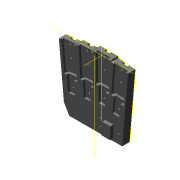
# Autodesk Inventor part: empty
Saved by Autodesk Inventor 2014 (Build 180170000, 170)
## iProperties
Created: 2015-04-13
Part Number: empty
Material: Generic
Document SubType Name: Modeling
Designer: Martin
Density: 1 g/cm^3
Appearance: Default
Author: Martin
Autodesk Inventor part; units mm, degrees
sketch "block_finger_attachment" plane through (0, 0, 0) normal (0, 0, 1) x (1, 0, 0)
  circle A0 centre (0, 0) radius 1.75
  circle A1 centre (0, -15) radius 1.75
  circle A2 centre (0, -46.8) radius 1.75
  line L0 (-8.5, -52.8) -> (8.5, -52.8)
  line L1 (8.5, -52.8) -> (8.5, 2.75)
  line L2 (8.5, 2.75) -> (-8.5, 2.75)
  line L3 (-8.5, 2.75) -> (-8.5, -52.8)
  line L4 (-8.5, -52.8) -> (8.5, 2.75) construction
  line L5 (8.5, -52.8) -> (-8.5, 2.75) construction
  line L6 (0, 2.75) -> (0, -52.8) construction
  line L7 (-8.5, -34.3) -> (8.5, -34.3)
  line L8 (-8.5, -31.5) -> (8.5, -31.5)
  line L9 (-4, -34.3) -> (-4, -52.8)
  line L10 (4, -34.3) -> (4, -52.8)
  line L11 (-8.5, -36.8) -> (8.5, -36.8) construction
  point P0 (0, -23.8707)
  point P1 (0, -25.025)
  dimension "d24" = 3.5
  dimension "d26" = 31.8
  dimension "d28" = 6
  dimension "d30" = 17
  dimension "d49" = 2.8
  dimension "d50" = 18.5
  dimension "d68" = 8
  dimension "d69" = 2.75
  dimension "d70" = 15
  dimension "d87" = 16
  measures "d24" diameter of A0
  measures "d26" distance of A2.centre A1.centre
  measures "d28" distance from line of L0 A2.centre
  measures "d30" distance of L0.start L0.end
  measures "d49" distance between parallel lines of L7 L8
  measures "d50" distance between parallel lines of L0 L7
  measures "d68" distance between parallel lines of L10 L9
  measures "d69" distance from line of L2 A0.centre
  measures "d70" distance of A0.centre A1.centre
  measures "d87" distance between parallel lines of L11 L0
sketch "block_finger_cutway" plane through (0, 0, 0) normal (0, 0, 1) x (1, 0, 0)
  circle A0 centre (0, 0) radius 1.75 construction
  circle A1 centre (0, -15) radius 1.75 construction
  circle A2 centre (0, -46.8) radius 1.75 construction
  line L0 (-8.5, -52.8) -> (8.5, -52.8) construction
  line L1 (8.5, -52.8) -> (8.5, 2.75) construction
  line L2 (8.5, 2.75) -> (-8.5, 2.75) construction
  line L3 (-8.5, 2.75) -> (-8.5, -52.8) construction
  line L4 (-8.5, -52.8) -> (8.5, 2.75) construction
  line L5 (8.5, -52.8) -> (-8.5, 2.75) construction
  line L6 (0, 2.75) -> (0, -52.8) construction
  line L7 (-8.5, -34.3) -> (8.5, -34.3) construction
  line L8 (-8.5, -31.5) -> (8.5, -31.5) construction
  line L9 (-4.5, -34.3) -> (-4.5, -52.8)
  line L10 (4.5, -34.3) -> (4.5, -52.8)
  line L11 (-8.5, -36.8) -> (8.5, -36.8) construction
  line L12 (-4.5, -52.8) -> (4.5, -52.8)
  line L13 (-4.5, -34.3) -> (-8, -34.3)
  line L14 (-8, -34.3) -> (-8, 2.75)
  line L15 (-8, 2.75) -> (8, 2.75)
  line L16 (8, 2.75) -> (8, -34.3)
  line L17 (4.5, -34.3) -> (8, -34.3)
  line L18 (4.5, -37.3) -> (8.5, -37.3)
  line L19 (8.5, -37.3) -> (8.5, -25.8)
  line L20 (8.5, -25.8) -> (8, -25.8)
  line L21 (-4.5, -52.8) -> (4.5, -52.8)
  line L22 (4.5, -52.8) -> (4.5, -53.8)
  line L23 (4.5, -53.8) -> (-4.5, -53.8)
  line L24 (-4.5, -53.8) -> (-4.5, -52.8)
  point P0 (0, -23.8707)
  point P1 (0, -25.025)
  dimension "d109" = 3.5
  dimension "d110" = 31.8
  dimension "d111" = 6
  dimension "d112" = 17
  dimension "d113" = 2.8
  dimension "d114" = 18.5
  dimension "d115" = 9
  dimension "d116" = 2.75
  dimension "d117" = 15
  dimension "d118" = 16
  dimension "d119" = 0.5
  dimension "d122" = 11.5
  dimension "d123" = 3
  dimension "d124" = 0.5
  dimension "d136" = 1
  measures "d109" diameter of A0
  measures "d110" distance of A2.centre A1.centre
  measures "d111" distance from line of L0 A2.centre
  measures "d112" distance of L0.start L0.end
  measures "d113" distance between parallel lines of L7 L8
  measures "d114" distance between parallel lines of L0 L7
  measures "d115" distance between parallel lines of L10 L9
  measures "d116" distance from line of L2 A0.centre
  measures "d117" distance of A0.centre A1.centre
  measures "d118" distance between parallel lines of L11 L0
  measures "d119" distance between parallel lines of L3 L14
  measures "d122" distance of L18.end L19.end
  measures "d123" distance between parallel lines of L7 L18
  measures "d124" distance between parallel lines of L16 L19
  measures "d136" distance between parallel lines of L0 L23
sketch "sk_main" plane through (0, 0, 0) normal (0, 1, 0) x (-1, 0, 0)
  line L0 (74.2951, 0) -> (-52.28, 0) projected
  line L1 (0, -108) -> (0, 18) projected
  line L2 (0, -3) -> (-23.2397, -3) construction
  line L3 (-8.5, -55.55) -> (-10.1097, -55.55) construction
  line L4 (0, -4) -> (22.6679, -4) construction
  line L5 (8.5, -55.55) -> (10.9991, -55.55) construction
  line L6 (0, -8) -> (45.2636, -8) construction
  line L7 (27.7608, -59.9653) -> (31.7206, -59.9653) construction
  line L8 (36.8027, -7.1853) -> (33.9128, -6.907)
  line L9 (33.9128, -6.907) -> (34.0419, -4.7972)
  line L10 (14.1837, -3.4811) -> (11.345, -3.293)
  line L11 (11.345, -3.293) -> (11.345, 0)
  line L12 (-14.772, -2.2592) -> (-11.642, -1.9853)
  line L13 (-11.642, -1.9853) -> (-11.642, 0)
  line L14 (56.2129, -9.0543) -> (49.5831, -77.9074)
  line L15 (42.6015, -90) -> (-26.6702, -90)
  line L16 (-26.6702, -90) -> (-34.1978, -3.9587)
  line L17 (-34.1978, -3.9587) -> (-31.7073, -3.7408)
  line L18 (49.5831, -77.9074) -> (42.6015, -90)
  line L19 (-8.5, 0) -> (-11.642, 0)
  line L20 (11.345, 0) -> (8.5, 0)
  line L21 (31.152, -4.5189) -> (34.0419, -4.7972)
  line L22 (53.7244, -8.8147) -> (56.2129, -9.0543)
  line L23 (33.9128, -6.907) -> (56.2129, -9.0543)
  line L24 (34.0419, -4.7972) -> (11.345, -3.293)
  line L25 (11.345, 0) -> (-11.642, 0)
  line L26 (-11.642, -1.9853) -> (-34.1978, -3.9587)
  circle A0 centre (-23, -5.7395) radius 1.75
  circle A1 centre (-21.6927, -20.6825) radius 1.75
  circle A2 centre (-18.9211, -52.3614) radius 1.75
  line L27 (-26.8658, -59.0794) -> (-9.9305, -57.5978)
  line L28 (-9.9305, -57.5978) -> (-14.772, -2.2592)
  line L29 (-14.772, -2.2592) -> (-31.7073, -3.7408)
  line L30 (-31.7073, -3.7408) -> (-26.8658, -59.0794)
  line L31 (-26.8658, -59.0794) -> (-14.772, -2.2592) construction
  line L32 (-9.9305, -57.5978) -> (-31.7073, -3.7408) construction
  line L33 (-23.2397, -3) -> (-18.3982, -58.3386) construction
  line L34 (-28.4782, -40.6498) -> (-11.5429, -39.1682)
  line L35 (-28.7222, -37.8605) -> (-11.7869, -36.3788)
  line L36 (-23.9953, -40.2576) -> (-22.383, -58.6872)
  line L37 (-16.0258, -39.5604) -> (-14.4134, -57.99)
  line L38 (-28.2603, -43.1403) -> (-11.325, -41.6587) construction
  circle A3 centre (0, -2.75) radius 1.75
  circle A4 centre (0, -17.75) radius 1.75
  circle A5 centre (0, -49.55) radius 1.75
  line L39 (-8.5, -55.55) -> (8.5, -55.55)
  line L40 (8.5, -55.55) -> (8.5, 0)
  line L41 (8.5, 0) -> (-8.5, 0)
  line L42 (-8.5, 0) -> (-8.5, -55.55)
  line L43 (-8.5, -55.55) -> (8.5, 0) construction
  line L44 (8.5, -55.55) -> (-8.5, 0) construction
  line L45 (0, 0) -> (0, -55.55) construction
  line L46 (-8.5, -37.05) -> (8.5, -37.05)
  line L47 (-8.5, -34.25) -> (8.5, -34.25)
  line L48 (-4, -37.05) -> (-4, -55.55)
  line L49 (4, -37.05) -> (4, -55.55)
  line L50 (-8.5, -39.55) -> (8.5, -39.55) construction
  circle A6 centre (22.5, -6.7449) radius 1.75
  circle A7 centre (21.5843, -21.7169) radius 1.75
  circle A8 centre (19.6429, -53.4576) radius 1.75
  line L51 (10.7925, -58.9275) -> (27.7608, -59.9653)
  line L52 (27.7608, -59.9653) -> (31.152, -4.5189)
  line L53 (31.152, -4.5189) -> (14.1837, -3.4811)
  line L54 (14.1837, -3.4811) -> (10.7925, -58.9275)
  line L55 (10.7925, -58.9275) -> (31.152, -4.5189) construction
  line L56 (27.7608, -59.9653) -> (14.1837, -3.4811) construction
  line L57 (22.6679, -4) -> (19.2766, -59.4464) construction
  line L58 (11.9219, -40.462) -> (28.8902, -41.4998)
  line L59 (12.0928, -37.6672) -> (29.0611, -38.705)
  line L60 (16.4135, -40.7367) -> (15.2841, -59.2022)
  line L61 (24.3986, -41.2251) -> (23.2692, -59.6906)
  line L62 (11.7693, -42.9573) -> (28.7376, -43.9951) construction
  circle A9 centre (45, -10.7373) radius 1.75
  circle A10 centre (43.5623, -25.6683) radius 1.75
  circle A11 centre (40.5144, -57.3219) radius 1.75
  line L63 (31.4785, -62.4796) -> (48.4002, -64.1089)
  line L64 (48.4002, -64.1089) -> (53.7244, -8.8147)
  line L65 (53.7244, -8.8147) -> (36.8027, -7.1853)
  line L66 (36.8027, -7.1853) -> (31.4785, -62.4796)
  line L67 (31.4785, -62.4796) -> (53.7244, -8.8147) construction
  line L68 (48.4002, -64.1089) -> (36.8027, -7.1853) construction
  line L69 (45.2636, -8) -> (39.9393, -63.2943) construction
  line L70 (33.2516, -44.0647) -> (50.1734, -45.6941)
  line L71 (33.52, -41.2776) -> (50.4417, -42.907)
  line L72 (37.7309, -44.496) -> (35.9578, -62.9109)
  line L73 (45.6941, -45.2628) -> (43.9209, -63.6776)
  line L74 (33.012, -46.5532) -> (49.9337, -48.1826) construction
  point P0 (0, 0)
  dimension "d32" = 23
  dimension "d37" = 22.5
  dimension "d41" = 22.5
  dimension "d31" = 5
  dimension "d33" = 3
  dimension "d34" = 1.6097
  dimension "d35" = 3.5
  dimension "d36" = 4
  dimension "d38" = 2.4991
  dimension "d39" = 5.5
  dimension "d40" = 8
  dimension "d42" = 3.9598
  dimension "d43" = 2.5
  dimension "d44" = 2.5
  dimension "d45" = 90
  constraints: 50 end point, 6 collinear, 6 parallel, 5 point on line, 4 perpendicular, 3 equal length, 1 vertical, 25 other
  measures "d33" distance between parallel lines of L0 L2
  measures "d34" distance of L3.start L3.end
  measures "d36" distance between parallel lines of L0 L4
  measures "d38" distance of L5.start L5.end
  measures "d40" distance between parallel lines of L0 L6
  measures "d42" distance of L7.start L7.end
  measures "d45" distance between parallel lines of L0 L15
extrude "ext_main" add sketch "sk_main" along normal blind 10 contours L11 L10 L54 L51 L52 L24 L9 L8 L66 L63 L64 L22 L14 L18 L15 L1 L39 L40 L0 | L40 L47 L1 A4 A3 L0 | L1 A3 A4 L47 L42 L0 | L40 L46 L1 L47 | L24 L52 L59 L54 | L42 L39 L1 L15 L16 L17 L30 L27 L28 L12 L13 L0 | L40 L39 L49 L46 | L1 L46 L42 L47 | L59 L52 L58 L54 | L49 L39 L1 A5 L46 | L1 A5 L39 L48 L46 | L58 L60 L51 L54 | L46 L48 L39 L42 | L52 L51 L61 L58 | L58 L61 L51 L60 | L28 L35 L30 L26 | L23 L64 L71 L66 | L28 L34 L30 L35 | L71 L64 L70 L66 | L28 L27 L37 L34 | L70 L72 L63 L66 | L34 L36 L27 L30 | L37 L27 L36 L34 | L64 L63 L73 L70 | L70 L73 L63 L72
ref_plane "plane_gear_4" through (-33.52, 0, -41.2776) normal (0.0958458, 0, -0.9953962) x (0, 1, 0)
ref_plane "plane_gear_3" through (-12.0928, 0, -37.6672) normal (0.0610485, 0, -0.9981348) x (0, 1, 0)
ref_plane "plane_gear_2" through (8.5, 0, -34.25) normal (0, 0, -1) x (-1, 0, 0)
ref_plane "plane_gear_1" through (28.7222, 0, -37.8605) normal (-0.0871557, 0, -0.9961947) x (0, -1, 0)
sketch "sk_cutways" plane through (0, 0, 0) normal (0, -1, 0) x (1, 0, 0)
  line L0 (0, -108) -> (0, 18) projected
  circle A0 centre (-45, -10.7373) radius 1.75 projected
  circle A1 centre (-43.5623, -25.6683) radius 1.75 projected
  circle A2 centre (-22.5, -6.7449) radius 1.75 projected
  circle A3 centre (-21.5843, -21.7169) radius 1.75 projected
  circle A4 centre (0, -17.75) radius 1.75 projected
  circle A5 centre (0, -2.75) radius 1.75 projected
  circle A6 centre (23, -5.7395) radius 1.75 projected
  circle A7 centre (21.6927, -20.6825) radius 1.75 projected
  circle A8 centre (-45, -10.7373) radius 1.75 construction
  circle A9 centre (-43.5623, -25.6683) radius 1.75 construction
  circle A10 centre (-40.5144, -57.3219) radius 1.75 construction
  line L1 (-48.4002, -64.1089) -> (-31.4785, -62.4796) construction
  line L2 (-31.4785, -62.4796) -> (-36.8027, -7.1853) construction
  line L3 (-36.8027, -7.1853) -> (-53.7244, -8.8147) construction
  line L4 (-53.7244, -8.8147) -> (-48.4002, -64.1089) construction
  line L5 (-48.4002, -64.1089) -> (-36.8027, -7.1853) construction
  line L6 (-31.4785, -62.4796) -> (-53.7244, -8.8147) construction
  line L7 (-45.2636, -8) -> (-39.9393, -63.2943) construction
  line L8 (-50.1734, -45.6941) -> (-33.2516, -44.0647) construction
  line L9 (-50.4417, -42.907) -> (-33.52, -41.2776) construction
  line L10 (-46.1918, -45.3107) -> (-44.4186, -63.7256)
  line L11 (-37.2332, -44.4481) -> (-35.4601, -62.863)
  line L12 (-49.9337, -48.1826) -> (-33.012, -46.5532) construction
  line L13 (-44.4186, -63.7256) -> (-35.4601, -62.863)
  line L14 (-46.1918, -45.3107) -> (-49.6757, -45.6462)
  line L15 (-49.6757, -45.6462) -> (-53.2267, -8.7668)
  line L16 (-53.2267, -8.7668) -> (-37.3004, -7.2332)
  line L17 (-37.3004, -7.2332) -> (-33.7493, -44.1127)
  line L18 (-37.2332, -44.4481) -> (-33.7493, -44.1127)
  line L19 (-36.9457, -47.4343) -> (-32.9641, -47.0509)
  line L20 (-32.9641, -47.0509) -> (-34.0663, -35.6039)
  line L21 (-34.0663, -35.6039) -> (-34.564, -35.6518)
  line L22 (-44.4186, -63.7256) -> (-35.4601, -62.863)
  line L23 (-35.4601, -62.863) -> (-35.3642, -63.8583)
  line L24 (-35.3642, -63.8583) -> (-44.3228, -64.721)
  line L25 (-44.3228, -64.721) -> (-44.4186, -63.7256)
  circle A11 centre (-22.5, -6.7449) radius 1.75 construction
  circle A12 centre (-21.5843, -21.7169) radius 1.75 construction
  circle A13 centre (-19.6429, -53.4576) radius 1.75 construction
  line L26 (-27.7608, -59.9653) -> (-10.7925, -58.9275) construction
  line L27 (-10.7925, -58.9275) -> (-14.1837, -3.4811) construction
  line L28 (-14.1837, -3.4811) -> (-31.152, -4.5189) construction
  line L29 (-31.152, -4.5189) -> (-27.7608, -59.9653) construction
  line L30 (-27.7608, -59.9653) -> (-14.1837, -3.4811) construction
  line L31 (-10.7925, -58.9275) -> (-31.152, -4.5189) construction
  line L32 (-22.6679, -4) -> (-19.2766, -59.4464) construction
  line L33 (-28.8902, -41.4998) -> (-11.9219, -40.462) construction
  line L34 (-29.0611, -38.705) -> (-12.0928, -37.6672) construction
  line L35 (-24.8976, -41.2556) -> (-23.7682, -59.7211)
  line L36 (-15.9144, -40.7062) -> (-14.785, -59.1717)
  line L37 (-28.7376, -43.9951) -> (-11.7693, -42.9573) construction
  line L38 (-23.7682, -59.7211) -> (-14.785, -59.1717)
  line L39 (-24.8976, -41.2556) -> (-28.3911, -41.4693)
  line L40 (-28.3911, -41.4693) -> (-30.653, -4.4884)
  line L41 (-30.653, -4.4884) -> (-14.6828, -3.5116)
  line L42 (-14.6828, -3.5116) -> (-12.421, -40.4925)
  line L43 (-15.9144, -40.7062) -> (-12.421, -40.4925)
  line L44 (-15.7313, -43.7006) -> (-11.7387, -43.4564)
  line L45 (-11.7387, -43.4564) -> (-12.4408, -31.9778)
  line L46 (-12.4408, -31.9778) -> (-12.9399, -32.0084)
  line L47 (-23.7682, -59.7211) -> (-14.785, -59.1717)
  line L48 (-14.785, -59.1717) -> (-14.724, -60.1698)
  line L49 (-14.724, -60.1698) -> (-23.7072, -60.7192)
  line L50 (-23.7072, -60.7192) -> (-23.7682, -59.7211)
  circle A14 centre (0, -2.75) radius 1.75 construction
  circle A15 centre (0, -17.75) radius 1.75 construction
  circle A16 centre (0, -49.55) radius 1.75 construction
  line L51 (-8.5, -55.55) -> (8.5, -55.55) construction
  line L52 (8.5, -55.55) -> (8.5, 0) construction
  line L53 (8.5, 0) -> (-8.5, 0) construction
  line L54 (-8.5, 0) -> (-8.5, -55.55) construction
  line L55 (-8.5, -55.55) -> (8.5, 0) construction
  line L56 (8.5, -55.55) -> (-8.5, 0) construction
  line L57 (0, 0) -> (0, -55.55) construction
  line L58 (-8.5, -37.05) -> (8.5, -37.05) construction
  line L59 (-8.5, -34.25) -> (8.5, -34.25) construction
  line L60 (-4.5, -37.05) -> (-4.5, -55.55)
  line L61 (4.5, -37.05) -> (4.5, -55.55)
  line L62 (-8.5, -39.55) -> (8.5, -39.55) construction
  line L63 (-4.5, -55.55) -> (4.5, -55.55)
  line L64 (-4.5, -37.05) -> (-8, -37.05)
  line L65 (-8, -37.05) -> (-8, 0)
  line L66 (-8, 0) -> (8, 0)
  line L67 (8, 0) -> (8, -37.05)
  line L68 (4.5, -37.05) -> (8, -37.05)
  line L69 (4.5, -40.05) -> (8.5, -40.05)
  line L70 (8.5, -40.05) -> (8.5, -28.55)
  line L71 (8.5, -28.55) -> (8, -28.55)
  line L72 (-4.5, -55.55) -> (4.5, -55.55)
  line L73 (4.5, -55.55) -> (4.5, -56.55)
  line L74 (4.5, -56.55) -> (-4.5, -56.55)
  line L75 (-4.5, -56.55) -> (-4.5, -55.55)
  circle A17 centre (23, -5.7395) radius 1.75 construction
  circle A18 centre (21.6927, -20.6825) radius 1.75 construction
  circle A19 centre (18.9211, -52.3614) radius 1.75 construction
  line L76 (9.9305, -57.5978) -> (26.8658, -59.0794) construction
  line L77 (26.8658, -59.0794) -> (31.7073, -3.7408) construction
  line L78 (31.7073, -3.7408) -> (14.772, -2.2592) construction
  line L79 (14.772, -2.2592) -> (9.9305, -57.5978) construction
  line L80 (9.9305, -57.5978) -> (31.7073, -3.7408) construction
  line L81 (26.8658, -59.0794) -> (14.772, -2.2592) construction
  line L82 (23.2397, -3) -> (18.3982, -58.3386) construction
  line L83 (11.5429, -39.1682) -> (28.4782, -40.6498) construction
  line L84 (11.7869, -36.3788) -> (28.7222, -37.8605) construction
  line L85 (15.5277, -39.5168) -> (13.9153, -57.9464)
  line L86 (24.4934, -40.3012) -> (22.8811, -58.7308)
  line L87 (11.325, -41.6587) -> (28.2603, -43.1403) construction
  line L88 (13.9153, -57.9464) -> (22.8811, -58.7308)
  line L89 (15.5277, -39.5168) -> (12.041, -39.2118)
  line L90 (12.041, -39.2118) -> (15.2701, -2.3028)
  line L91 (15.2701, -2.3028) -> (31.2092, -3.6972)
  line L92 (31.2092, -3.6972) -> (27.9801, -40.6063)
  line L93 (24.4934, -40.3012) -> (27.9801, -40.6063)
  line L94 (24.232, -43.2898) -> (28.2167, -43.6384)
  line L95 (28.2167, -43.6384) -> (29.219, -32.1822)
  line L96 (29.219, -32.1822) -> (28.7209, -32.1386)
  line L97 (13.9153, -57.9464) -> (22.8811, -58.7308)
  line L98 (22.8811, -58.7308) -> (22.7939, -59.727)
  line L99 (22.7939, -59.727) -> (13.8281, -58.9426)
  line L100 (13.8281, -58.9426) -> (13.9153, -57.9464)
  constraints: 9 other
extrude "ext_cut_linactcutways" cut sketch "sk_cutways" against normal blind 3 contours L74 L75 L63 L0 | L0 L63 L73 L74 | L63 L60 L64 L65 L66 L0 A5 A4 | L0 A4 A5 L66 L67 L68 L61 L63 | L61 L68 L67 L71 L70 L69 | L14 L15 L16 L17 L18 L11 L13 L10 | L13 L23 L24 L25 | L11 L18 L17 L21 L20 L19 | L39 L40 L41 L42 L43 L36 L38 L35 | L38 L48 L49 L50 | L36 L43 L42 L46 L45 L44 | L89 L90 L91 L92 L93 L86 L88 L85 | L88 L98 L99 L100 | L86 L93 L92 L96 L95 L94
chamfer "chamfer_linact_side" distance 1 angle 45 4 edges at (-33.5152, 0, -41.3274) (-12.0898, 0, -37.7171) (8.5, 0, -34.3) (28.7179, 0, -37.9103)
sketch "Sketch5" plane through (-33.52, 0, -41.2776) normal (0.0958458, 0, -0.9953962) x (0, 1, 0)
  line L0 (0, 0) -> (0, -17) projected
  line L1 (0, 0) -> (0, -17)
  line L2 (0, -17) -> (3, -17)
  line L3 (3, -17) -> (3, 0)
  line L4 (3, 0) -> (0, 0)
  arc A0 (3, -17) -> (3, 0) centre (-0.0208, -8.5) ccw
  line L5 (3, -8.5) -> (9, -8.5) construction
  point P0 (0, 37.322)
  dimension "d134" = 6
  dimension "d135" = 3
  constraints: 10 end point, 3 equal length, 3 point on circle, 1 centre point, 1 midpoint, 1 perpendicular
  measures "d134" distance of L5.start L5.end
  measures "d135" distance of L3.end L0.start
extrude "ext_cut_gear_4" cut sketch "Sketch5" along normal up to surface (2.8 mm away)
sketch "Sketch6" plane through (-12.0928, 0, -37.6672) normal (0.0610485, 0, -0.9981348) x (0, 1, 0)
  line L0 (0, 0) -> (0, -17) projected
  line L1 (0, -17) -> (0, 0)
  line L2 (0, 0) -> (3, 0)
  line L3 (3, 0) -> (3, -17)
  line L4 (3, -17) -> (0, -17)
  arc A0 (3, -17) -> (3, 0) centre (-0.0208, -8.5) ccw
  line L5 (3, -8.5) -> (9, -8.5)
  point P0 (0, 14.3698)
  dimension "d132" = 6
  dimension "d133" = 3
  constraints: 10 end point, 3 parallel, 3 point on circle, 1 centre point, 1 collinear, 1 midpoint, 1 perpendicular
  measures "d132" distance of L5.start L5.end
  measures "d133" distance of L0.start L2.end
extrude "ext_cut_gear_3" cut sketch "Sketch6" along normal up to surface (2.8 mm away)
sketch "Sketch7" plane through (8.5, 0, -34.25) normal (0, 0, -1) x (-1, 0, 0)
  line L0 (0, 0) -> (17, 0) projected
  line L1 (0, 0) -> (17, 0)
  line L2 (17, 0) -> (17, 3)
  line L3 (17, 3) -> (0, 3)
  line L4 (0, 3) -> (0, 0)
  arc A0 (17, 3) -> (0, 3) centre (8.5, -0.0208) ccw
  line L5 (8.5, 9) -> (8.5, 3) construction
  point P0 (8.5, 0)
  dimension "d130" = 6
  dimension "d131" = 3
  constraints: 10 end point, 3 equal length, 3 point on circle, 1 centre point, 1 midpoint, 1 perpendicular
  measures "d130" distance of L5.start L5.end
  measures "d131" distance of L0.end L2.end
extrude "ext_cut_gear_2" cut sketch "Sketch7" along normal up to surface (2.8 mm away)
sketch "Sketch8" plane through (28.7222, 0, -37.8605) normal (-0.0871557, 0, -0.9961947) x (0, -1, 0)
  line L0 (0, 0) -> (0, 17) projected
  line L1 (0, 17) -> (0, 0)
  line L2 (0, 0) -> (-3, 0)
  line L3 (-3, 0) -> (-3, 17)
  line L4 (-3, 17) -> (0, 17)
  arc A0 (-3, 17) -> (-3, 0) centre (0.0208, 8.5) ccw
  line L5 (-9, 8.5) -> (-3, 8.5) construction
  point P0 (0, 31.9127)
  dimension "d128" = 3
  dimension "d129" = 6
  constraints: 10 end point, 3 equal length, 3 point on circle, 1 centre point, 1 midpoint, 1 perpendicular
  measures "d128" distance of L3.end L0.end
  measures "d129" distance of L5.start L5.end
extrude "ext_cut_gear_1" cut sketch "Sketch8" along normal up to surface (2.8 mm away)
sketch "sk_thumb_axis" plane through (0, 0, 0) normal (0, 0, 1) x (1, 0, 0)
  line L0 (-2, 0) -> (12, 0) projected
  line L1 (0, -24) -> (0, 4) projected
  point P0 (0, 0)
  point P1 (10, -20)
  dimension "d66" = 20
  dimension "d67" = 10
  measures "d66" distance from line of L0 point (10, -20)
  measures "d67" distance from line of L1 point (10, -20)
ref_plane "plane_thumblinact" through (-9, 0, 0) normal (1, 0, 0) x (0, 1, 0)
sketch "Sketch9" plane through (0, 10, 0) normal (0, 1, 0) x (1, 0, 0)
  circle A0 centre (-40.5144, 57.3219) radius 1.75 projected
  circle A1 centre (-43.5623, 25.6683) radius 1.75 projected
  circle A2 centre (-45, 10.7373) radius 1.75 projected
  circle A3 centre (0, 49.55) radius 1.75 projected
  circle A4 centre (0, 17.75) radius 1.75 projected
  circle A5 centre (0, 2.75) radius 1.75 projected
  circle A6 centre (18.9211, 52.3614) radius 1.75 projected
  circle A7 centre (21.6927, 20.6825) radius 1.75 projected
  circle A8 centre (23, 5.7395) radius 1.75 projected
  circle A9 centre (-19.6429, 53.4576) radius 1.75 projected
  circle A10 centre (-21.5843, 21.7169) radius 1.75 projected
  circle A11 centre (-22.5, 6.7449) radius 1.75 projected
  line L0 (11.642, 1.9853) -> (34.1978, 3.9587) projected
  line L1 (-56.2129, 9.0543) -> (-33.9128, 6.907) projected
  line L2 (-34.0419, 4.7972) -> (-11.345, 3.293) projected
  line L3 (-11.345, 0) -> (11.642, 0) projected
  circle A12 centre (-40.5144, 57.3219) radius 3.25
  circle A13 centre (-19.6429, 53.4576) radius 3.25
  circle A14 centre (0, 49.55) radius 3.25
  circle A15 centre (18.9211, 52.3614) radius 3.25
  circle A16 centre (21.6927, 20.6825) radius 3.25
  circle A17 centre (23, 5.7395) radius 3.25
  circle A18 centre (0, 17.75) radius 3.25
  circle A19 centre (-21.5843, 21.7169) radius 3.25
  circle A20 centre (-22.5, 6.7449) radius 3.25
  circle A21 centre (0, 2.75) radius 3.25
  circle A22 centre (-43.5623, 25.6683) radius 3.25
  circle A23 centre (-45, 10.7373) radius 3.25
  line L4 (-48.4986, 8.3115) -> (-48.235, 11.0488)
  line L5 (-42.0285, 7.6885) -> (-41.765, 10.4258)
  line L6 (-25.9219, 4.259) -> (-25.7429, 6.9598)
  line L7 (-19.4361, 3.8292) -> (-19.2571, 6.53)
  line L8 (-3.25, 0) -> (-3.25, 2.75)
  line L9 (3.25, 0) -> (3.25, 2.75)
  line L10 (20.002, 2.7167) -> (19.7624, 5.4563)
  line L11 (26.4773, 3.2833) -> (26.2376, 6.0228)
  circle A24 centre (-40.5144, 57.3219) radius 1.75 projected
  circle A25 centre (-43.5623, 25.6683) radius 1.75 projected
  circle A26 centre (-45, 10.7373) radius 1.75 projected
  circle A27 centre (0, 49.55) radius 1.75 projected
  circle A28 centre (0, 17.75) radius 1.75 projected
  circle A29 centre (0, 2.75) radius 1.75 projected
  circle A30 centre (18.9211, 52.3614) radius 1.75 projected
  circle A31 centre (21.6927, 20.6825) radius 1.75 projected
  circle A32 centre (23, 5.7395) radius 1.75 projected
  circle A33 centre (-19.6429, 53.4576) radius 1.75 projected
  circle A34 centre (-21.5843, 21.7169) radius 1.75 projected
  circle A35 centre (-22.5, 6.7449) radius 1.75 projected
  line L12 (11.642, 0) -> (11.642, 1.9853) projected
  line L13 (11.642, 1.9853) -> (34.1978, 3.9587) projected
  line L14 (34.1978, 3.9587) -> (26.6702, 90) projected
  line L15 (26.6702, 90) -> (-42.6015, 90) projected
  line L16 (-42.6015, 90) -> (-49.5831, 77.9074) projected
  line L17 (-49.5831, 77.9074) -> (-56.2129, 9.0543) projected
  line L18 (-56.2129, 9.0543) -> (-33.9128, 6.907) projected
  line L19 (-33.9128, 6.907) -> (-34.0419, 4.7972) projected
  line L20 (-34.0419, 4.7972) -> (-11.345, 3.293) projected
  line L21 (-11.345, 3.293) -> (-11.345, 0) projected
  line L22 (-11.345, 0) -> (11.642, 0) projected
  point P0 (0, 0)
  dimension "d63" = 6.5
  constraints: 16 end point, 12 centre point, 12 coincident, 11 equal radius, 8 perpendicular, 8 point on circle, 8 point on line, 8 tangent
  measures "d63" diameter of A15
extrude "ext_cut_backscrewheads" cut sketch "Sketch9" against normal blind 3 contours L10 A17 L0 | A17 L0 | L3 A21 L9 | A17 L11 L0 | L3 A21 | L3 L8 A21 | L2 A20 L7 | L2 A20 | L4 A23 L1 | L2 L6 A20 | A23 L1 | A23 L5 L1 | A12 | A13 | A14 | A15 | A16 | A18 | A19 | A22 picked at (23.2301, 3.3341) picked at (0.0703, 0.3376) picked at (-22.6896, 4.3653) picked at (-45.246, 8.3333)
sketch "Sketch19" plane through (0, 0, 0) normal (0, -1, 0) x (1, 0, 0)
  line L0 (26.6702, -90) -> (-42.6015, -90) projected
  line L1 (10, -108) -> (10, 18) projected
  line L2 (4.5, -86.5) -> (15.5, -86.5)
  line L3 (15.5, -86.5) -> (15.5, -71)
  line L4 (15.5, -71) -> (4.5, -71)
  line L5 (4.5, -71) -> (4.5, -86.5)
  line L6 (4.5, -86.5) -> (15.5, -71) construction
  line L7 (15.5, -86.5) -> (4.5, -71) construction
  point P0 (0, 0)
  point P1 (10, -78.75)
  dimension "d137" = 3.5
  dimension "d138" = 15.5
  dimension "d139" = 11
  constraints: 12 end point, 2 midpoint, 2 parallel, 1 horizontal, 1 perpendicular, 1 point on line
  measures "d137" distance between parallel lines of L0 L2
  measures "d138" distance of L2.end L3.end
  measures "d139" distance between parallel lines of L3 L5
ref_plane "Work Plane12" through (4.2, -4.55, -91.2779) normal (0, 1, 0) x (0, 0, 1)
extrude "Extrusion16" add sketch "Sketch19" along normal up to surface (4.55 mm away)
sketch "Sketch20" plane through (15.5, 0, -86.5) normal (0, 0, -1) x (-1, 0, 0)
  line L0 (11, -4.55) -> (0, -4.55) projected
  line L1 (0, 0) -> (11, 0) projected
  line L2 (5.5, 0) -> (5.5, -4.55) construction
  circle A0 centre (5.5, -2.5) radius 1
  point P0 (15.5, 0)
  dimension "d142" = 2
  dimension "d143" = 2.5
  constraints: 2 end point, 2 midpoint, 1 centre point, 1 point on line
  measures "d142" diameter of A0
  measures "d143" distance from line of L1 A0.centre
extrude "Extrusion17" cut sketch "Sketch20" against normal blind 8
sketch "sk_thumbscrews" plane through (0, 10, 0) normal (0, 1, 0) x (1, 0, 0)
  circle A0 centre (18.9211, 52.3614) radius 3.25 projected
  circle A1 centre (-2.3, 81.5) radius 1.5
  circle A2 centre (-2.3, 71.5) radius 1.5
  line L0 (26.2376, 6.0228) -> (26.4773, 3.2833) projected
  line L1 (26.4773, 3.2833) -> (34.1978, 3.9587) projected
  line L2 (34.1978, 3.9587) -> (26.6702, 90) projected
  line L3 (26.6702, 90) -> (-42.6015, 90) projected
  line L4 (-42.6015, 90) -> (-49.5831, 77.9074) projected
  line L5 (-49.5831, 77.9074) -> (-56.2129, 9.0543) projected
  line L6 (-56.2129, 9.0543) -> (-48.4986, 8.3115) projected
  line L7 (-48.4986, 8.3115) -> (-48.235, 11.0488) projected
  arc A3 (-41.765, 10.4258) -> (-48.235, 11.0488) centre (-45, 10.7373) ccw projected
  line L8 (-41.765, 10.4258) -> (-42.0285, 7.6885) projected
  line L9 (-42.0285, 7.6885) -> (-33.9128, 6.907) projected
  line L10 (-33.9128, 6.907) -> (-34.0419, 4.7972) projected
  line L11 (-34.0419, 4.7972) -> (-25.9219, 4.259) projected
  line L12 (-25.9219, 4.259) -> (-25.7429, 6.9598) projected
  arc A4 (-19.2571, 6.53) -> (-25.7429, 6.9598) centre (-22.5, 6.7449) ccw projected
  line L13 (-19.2571, 6.53) -> (-19.4361, 3.8292) projected
  line L14 (-19.4361, 3.8292) -> (-11.345, 3.293) projected
  line L15 (-11.345, 3.293) -> (-11.345, 0) projected
  line L16 (-11.345, 0) -> (-3.25, 0) projected
  line L17 (-3.25, 0) -> (-3.25, 2.75) projected
  arc A5 (3.25, 2.75) -> (-3.25, 2.75) centre (0, 2.75) ccw projected
  line L18 (3.25, 2.75) -> (3.25, 0) projected
  line L19 (3.25, 0) -> (11.642, 0) projected
  line L20 (11.642, 0) -> (11.642, 1.9853) projected
  line L21 (11.642, 1.9853) -> (20.002, 2.7167) projected
  line L22 (20.002, 2.7167) -> (19.7624, 5.4563) projected
  arc A6 (26.2376, 6.0228) -> (19.7624, 5.4563) centre (23, 5.7395) ccw projected
  circle A7 centre (-43.5623, 25.6683) radius 3.25 projected
  circle A8 centre (0, 17.75) radius 3.25 projected
  circle A9 centre (18.9211, 52.3614) radius 3.25 projected
  circle A10 centre (-19.6429, 53.4576) radius 3.25 projected
  circle A11 centre (-40.5144, 57.3219) radius 3.25 projected
  circle A12 centre (0, 49.55) radius 3.25 projected
  circle A13 centre (21.6927, 20.6825) radius 3.25 projected
  circle A14 centre (-21.5843, 21.7169) radius 3.25 projected
  circle A15 centre (22.3, 77.35) radius 1.5
  circle A16 centre (-2.3, 81.5) radius 3.25
  circle A17 centre (-2.3, 71.5) radius 3.25
  circle A18 centre (22.3, 77.35) radius 3.25
  point P0 (0, 0)
  constraints: 6 centre point, 3 coincident, 3 equal radius, 6 other
extrude "ext_cut_thumbfixscrews" cut sketch "sk_thumbscrews" against normal through all contours A1 | A2 | A15
extrude "ext_cut_thumbfixscrews_heads" cut sketch "sk_thumbscrews" against normal up to surface (3 mm away) contours A16 | A17 | A18
equation "\"d66\" = palm_thumb_x_offset"
equation "\"d67\" = palm_thumb_y_offset"
equation "\"model_linactgear_housing_depth\" = 6"
equation "\"model_linact_cutway_depth\" = 3"
equation "\"palm_thumb_x_offset\" = 20"
equation "\"palm_thumb_y_offset\" = 10"
body "Solid2"
